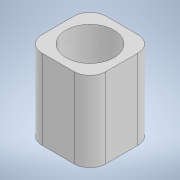
# Autodesk Inventor part: SpacerBlock_25mm
Saved by Autodesk Inventor 2021 (Build 250183000, 183)
## iProperties
Created: 2021-10-18
Part Number: SpacerBlock_25mm
Material: Generic
Document SubType Name: Modeling
Designer: Jorian Bruslind
Density: 1 g/cm^3
Appearance: Default
Author: Jorian Bruslind
Autodesk Inventor part; units mm, degrees
ref_plane "YZ Plane" through (0, 0, 0) normal (1, 0, 0) x (0, 1, 0)
ref_plane "XZ Plane" through (0, 0, 0) normal (0, 1, 0) x (-1, 0, 0)
ref_plane "XY Plane" through (0, 0, 0) normal (0, 0, 1) x (1, 0, 0)
sketch "Sketch1" plane through (0, 0, 0) normal (0, 1, 0) x (-1, 0, 0)
  line L0 (0, 0) -> (20, 0)
  line L1 (20, 0) -> (20, -20)
  line L2 (20, -20) -> (0, -20)
  line L3 (0, -20) -> (0, 0)
  dimension "d0" = 20
  dimension "d1" = 20
  constraints: 8 end point, 2 parallel, 1 horizontal, 1 perpendicular
  measures "d0" distance of L1.end L2.end
  measures "d1" distance of L0.end L1.end
extrude "Extrusion1" add sketch "Sketch1" along normal blind 25
sketch "Sketch2" plane through (0, 25, 0) normal (0, 1, 0) x (1, 0, 0)
  circle A0 centre (-10, 10) radius 3
  line L0 (0, 20) -> (-20, 20) projected
  line L1 (-20, 20) -> (-20, 0) projected
  point P0 (0, 0)
  dimension "d4" = 6
  dimension "d5" = 10
  dimension "d6" = 10
  constraints: 1 centre point
  measures "d4" diameter of A0
  measures "d5" distance from line of L0 A0.centre
  measures "d6" distance from line of L1 A0.centre
extrude "Extrusion2" cut sketch "Sketch2" against normal through all
fillet "Fillet1" radius 5 4 edges at (-20, 12.5, -20) (0, 12.5, 0) (0, 12.5, -20) (-20, 12.5, 0)
sketch "Sketch3" plane through (0, 25, 0) normal (0, 1, 0) x (1, 0, 0)
  circle A0 centre (-10, 10) radius 3 projected
  circle A1 centre (-10, 10) radius 7.5
  point P0 (0, 0)
  dimension "d10" = 15
  constraints: 1 centre point, 1 coincident
  measures "d10" diameter of A1
extrude "Extrusion3" cut sketch "Sketch3" against normal blind 19
body "Solid1"
